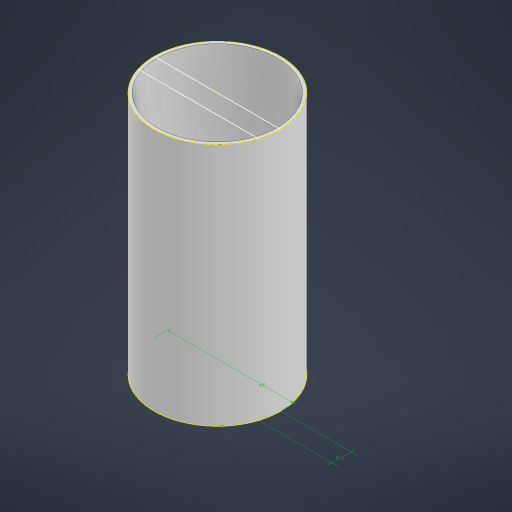
# Autodesk Inventor part: Tank_M2
Saved by Autodesk Inventor 2023 (Build 270158000, 158)
## iProperties
Created: 2022-08-20
Part Number: Tank_M2
Material: Generic
Document SubType Name: Modeling
Designer: Mike
Density: 1 g/cm^3
Appearance: Default
Author: Mike
Autodesk Inventor part; units mm, degrees
ref_plane "YZ Plane" through (0, 0, 0) normal (1, 0, 0) x (0, 1, 0)
ref_plane "XZ Plane" through (0, 0, 0) normal (0, 1, 0) x (-1, 0, 0)
ref_plane "XY Plane" through (0, 0, 0) normal (0, 0, 1) x (1, 0, 0)
sketch "Sketch1" plane through (0, 0, 0) normal (0, 1, 0) x (-1, 0, 0)
  circle A0 centre (0, 0) radius 200
  circle A1 centre (0, 0) radius 210
  dimension "d0" = 400
  dimension "d1" = 420
  constraints: 2 centre point, 2 coincident
  measures "d0" diameter of A0
  measures "d1" diameter of A1
extrude "Extrusion1" add sketch "Sketch1" against normal blind 10 contours A0 | A1
extrude "Extrusion2" add sketch "Sketch1" along normal blind 800
sketch "Sketch4" plane through (0, -10, 0) normal (0, -1, 0) x (1, 0, 0)
  circle A0 centre (0, 0) radius 210 projected
  line L0 (210, 0) -> (-210, 0)
  line L1 (200.1693, 63.5) -> (-200.1693, 63.5)
  dimension "d25" = 420
  dimension "d26" = 63.5
  constraints: 4 end point, 4 point on circle, 2 horizontal
  measures "d25" distance of L0.start L0.end
  measures "d26" distance between parallel lines of L1 L0
sketch "Sketch5" plane through (0, 800, 0) normal (0, 1, 0) x (1, 0, 0)
  circle A0 centre (0, 0) radius 210 projected
  line L0 (-210, 0) -> (210, 0)
  line L1 (-200.1693, -63.5) -> (200.1693, -63.5)
  dimension "d27" = 420
  dimension "d29" = 63.5
  constraints: 4 end point, 4 point on circle, 2 horizontal
  measures "d27" distance of L0.start L0.end
  measures "d29" distance between parallel lines of L1 L0
body "Solid1"
